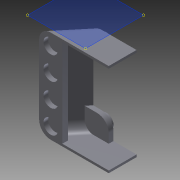
# Autodesk Inventor part: LEGO Brick Window
Saved by Autodesk Inventor 2011 SP1 (Build 150282100, 282)
## iProperties
Company: Allseas Engineering BV
Created: 2011-09-28
Part Number: LEGO Brick Window
Cost Center: 0 kg
Material: Steel
Document SubType Name: Modeling
Designer: BvH
Authority: 0 mm^3
Stock Number: =<Filenr>_<Document number>
Density: 7.85 g/cm^3
Act. Code: DW000
SaveDate: 2011-07-28
SaveTime: 18:32
FileName: Standard
TotalMass: 0 kg
TotalVolume: 0 mm^3
Subject: =<Title><TITLE 1_2> <TITLE 2_2>
Author: BvH
Autodesk Inventor part; units mm, degrees
ref_plane "YZ Plane" through (0, 0, 0) normal (1, 0, 0) x (0, 1, 0)
ref_plane "XY Plane" through (0, 0, 0) normal (0, 0, 1) x (1, 0, 0)
ref_plane "Work Plane1" through (0, 12.8, 0) normal (0, 1, 0) x (-1, 0, 0)
sketch "Sketch5" plane through (0, 12.8, 0) normal (0, 1, 0) x (-1, 0, 0)
  line L0 (12, -16) -> (0, -16)
  line L1 (0, -16) -> (0, 16)
  line L2 (0, 16) -> (12, 16)
  arc A0 (16, 12) -> (12, 16) centre (12, 12) ccw
  line L3 (16, 12) -> (16, -12)
  arc A1 (12, -16) -> (16, -12) centre (12, -12) ccw
  line L4 (8, -16) -> (8, -12)
  arc A2 (12, -8) -> (8, -12) centre (12, -12) ccw
  line L5 (12, -8) -> (16, -8)
  line L6 (16, -8) -> (8, -16) construction
  line L7 (16, 8) -> (12, 8)
  line L8 (8, 12) -> (8, 16)
  line L9 (16, 8) -> (8, 16) construction
  arc A3 (8, 12) -> (12, 8) centre (12, 12) ccw
  point P0 (0, 0)
  point P1 (0, 0)
  dimension "d23" = 32
  dimension "d24" = 16
  dimension "d25" = 4
  dimension "d40" = 8
  constraints: 20 end point, 8 point on circle, 7 tangent, 4 centre point, 4 horizontal, 4 point on line, 4 vertical, 3 equal length, 3 midpoint, 1 coincident, 1 collinear, 1 equal radius
  measures "d23" distance between parallel lines of L2 L0
  measures "d24" distance between parallel lines of L1 L3
  measures "d25" radius of A1
  measures "d40" distance between parallel lines of L4 L3
sketch "Sketch6" plane through (0, 0, 0) normal (0, 1, 0) x (-1, 0, 0)
  line L0 (0, -16) -> (0, 16) projected
  line L1 (0, 16) -> (20, 16)
  arc A0 (24, 12) -> (20, 16) centre (20, 12) ccw
  line L2 (0, -16) -> (20, -16)
  arc A1 (20, -16) -> (24, -12) centre (20, -12) ccw
  line L3 (24, -12) -> (24, 12)
  line L4 (16, 16) -> (16, -16)
  dimension "d26" = 4
  dimension "d27" = 24
  dimension "d35" = 8
  constraints: 8 end point, 4 point on circle, 4 tangent, 2 centre point, 2 horizontal, 2 point on line, 2 vertical, 1 equal radius
  measures "d26" radius of A1
  measures "d27" distance between parallel lines of L0 L3
  measures "d35" distance between parallel lines of L4 L3
loft "Loft1" add profiles "Sketch5", "Sketch6"
shell "Shell2" thickness 0.8 removed faces 3 at (-5.3333, 12.8, 4) at (0, 8.5333, 5.3333) at (-8, 0, 4)
ref_plane "Work Plane2" through (0, 2, 0) normal (0, 1, 0) x (-1, 0, 0)
sketch "Sketch7" plane through (0, 2, 0) normal (0, 1, 0) x (-1, 0, 0)
  line L0 (18.75, -16) -> (0, -16) projected
  line L1 (0, 15.2) -> (0, 16) projected
  line L2 (0, 16) -> (18.75, 16) projected
  arc A0 (22.75, 12) -> (18.75, 16) centre (18.75, 12) ccw projected
  line L3 (22.75, 12) -> (22.75, -12) projected
  arc A1 (18.75, -16) -> (22.75, -12) centre (18.75, -12) ccw projected
  line L4 (18.75, -16) -> (0, -16) projected
  line L5 (0, 15.2) -> (0, 16) projected
  line L6 (0, 16) -> (18.75, 16) projected
  line L7 (24, -12) -> (24, 12) construction
  line L8 (0, -15.2) -> (18.75, -15.2) projected
  arc A2 (18.75, -15.2) -> (21.8066, -12) centre (21.8066, -12) ccw projected
  line L9 (21.8066, -12) -> (21.8066, 12) projected
  arc A3 (21.8066, 12) -> (18.75, 15.2) centre (18.75, 15.2) ccw projected
  line L10 (18.75, 15.2) -> (0, 15.2) projected
  line L11 (0, -16) -> (0, -15.2) projected
  line L12 (0, -15.2) -> (18.75, -15.2) projected
  arc A4 (18.75, -15.2) -> (21.8066, -12) centre (21.8066, -12) ccw projected
  line L13 (21.8066, -12) -> (21.8066, 12) projected
  arc A5 (21.8066, 12) -> (18.75, 15.2) centre (18.75, 15.2) ccw projected
  line L14 (18.75, 15.2) -> (0, 15.2) projected
  line L15 (0, -16) -> (0, -15.2) projected
  line L16 (16, 16) -> (16, -16) projected
  arc A6 (22.75, 12) -> (18.75, 16) centre (18.75, 12) ccw projected
  line L17 (22.75, 12) -> (22.75, -12) projected
  arc A7 (18.75, -16) -> (22.75, -12) centre (18.75, -12) ccw projected
  constraints: 4 other
loft "Loft2" add profiles "Sketch7", "Sketch6" contours L0 L16 L8 A2 A1 | A2 L8 L16 L10 A3 A0 L9 A1 | A2 L9 A3 A0 L3 A1 | L16 L2 A0 A3 L10 / L4 L1 A0 L3 A1 L2
ref_plane "Work Plane3" through (0, 11.2, 0) normal (0, 1, 0) x (-1, 0, 0)
sketch "Sketch8" plane through (0, 11.2, 0) normal (0, 1, 0) x (-1, 0, 0)
  line L0 (13, -16) -> (0, -16) projected
  line L1 (0, -16) -> (0, -15.2) construction
  line L2 (0, -15.2) -> (13, -15.2) construction
  arc A0 (13, -15.2) -> (16.0566, -12) centre (16.0566, -12) ccw construction
  line L3 (16.0566, -12) -> (16.0566, 12) construction
  arc A1 (16.0566, 12) -> (13, 15.2) centre (13, 15.2) ccw construction
  line L4 (13, 15.2) -> (0, 15.2) construction
  line L5 (0, 15.2) -> (0, 16) construction
  line L6 (0, 16) -> (13, 16) projected
  arc A2 (17, 12) -> (13, 16) centre (13, 12) ccw projected
  line L7 (17, 12) -> (17, -12) projected
  arc A3 (13, -16) -> (17, -12) centre (13, -12) ccw projected
  line L8 (8, -16) -> (8, -12) projected
  arc A4 (12, -8) -> (8, -12) centre (12, -12) ccw projected
  arc A5 (8, 12) -> (12, 8) centre (12, 12) ccw projected
  line L9 (8, 12) -> (8, 16) projected
  line L10 (12, -8) -> (17, -8)
  line L11 (12, 8) -> (17, 8)
  constraints: 4 end point, 2 horizontal, 2 point on line, 2 tangent, 2 other
loft "Loft3" add profiles "Sketch5", "Sketch8" contours L0 L4 A2 L5 L3 A1 / L0 L8 A4 L10 L7 A3
loft "Loft4" add profiles "Sketch5", "Sketch8" contours L7 A3 L8 L2 A0 L3 / L6 A2 L7 L11 A5 L9
sketch "Sketch9" plane through (-12, 12.8, 16) normal (0, 1, 0) x (1, 0, 0)
  arc A0 (0, 24) -> (4, 28) centre (0, 28) ccw construction
  arc A1 (4, 4) -> (0, 8) centre (0, 4) ccw construction
  circle A2 centre (0, 4) radius 2.5
  circle A3 centre (0, 28) radius 2.5
  dimension "d51" = 5
  constraints: 2 centre point, 2 coincident, 1 equal radius
  measures "d51" diameter of A3
extrude "Extrusion5" add sketch "Sketch9" along normal blind 1.6 separate body
shell "Shell3" thickness 0.8 removed faces 2 at (-12.6238, 14.4, 10.9942) at (-12.6238, 14.4, -11.4474) bodies 2
sketch "Sketch10" plane through (-20, 0, 16) normal (0, -1, 0) x (1, 0, 0)
  line L0 (-4, -28) -> (-4, -4) construction
  line L1 (-8.8, -16) -> (24.8, -16) construction
  line L2 (0, -4) -> (0, -28) construction
  circle A0 centre (0, -4) radius 2.5
  circle A1 centre (0, -12) radius 2.5
  circle A2 centre (0, -20) radius 2.5
  circle A3 centre (0, -28) radius 2.5
  point P0 (0, -16)
  dimension "d55" = 4
  dimension "d56" = 24
  dimension "d57" = 5
  dimension "d58" = 8
  dimension "d59" = 8
  constraints: 4 centre point, 3 equal radius, 3 point on line, 2 coincident, 2 end point, 1 midpoint, 1 vertical
  measures "d55" distance between parallel lines of L0 L2
  measures "d56" distance of L2.start L2.end
  measures "d57" diameter of A0
  measures "d58" distance of A1.centre A0.centre
  measures "d59" distance of A3.centre A2.centre
extrude "Extrusion6" cut sketch "Sketch10" against normal blind 1.6 bodies 1
body "Solid1"
body "Solid3"
body "Solid4"
